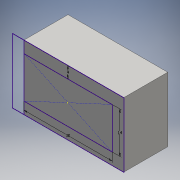
# Autodesk Inventor part: Solenoid Mount
Saved by Autodesk Inventor 2016 (Build 200138000, 138)
## iProperties
Created: 2016-05-08
Part Number: Solenoid Mount
Material: Generic
Document SubType Name: Modeling
Designer: Kenneth Daniel
Density: 1 g/cm^3
Appearance: Default
Author: Kenneth Daniel
Autodesk Inventor part; units mm, degrees
ref_plane "YZ Plane" through (0, 0, 0) normal (1, 0, 0) x (0, 1, 0)
ref_plane "XZ Plane" through (0, 0, 0) normal (0, 1, 0) x (-1, 0, 0)
ref_plane "XY Plane" through (0, 0, 0) normal (0, 0, 1) x (1, 0, 0)
sketch "Sketch1" plane through (0, 0, 0) normal (0, 1, 0) x (-1, 0, 0)
  line L0 (-15, 7) -> (-15, -7)
  line L1 (-15, -7) -> (15, -7)
  line L2 (15, -7) -> (15, 7)
  line L3 (15, 7) -> (-15, 7)
  line L4 (-15, 7) -> (15, -7) construction
  line L5 (-15, -7) -> (15, 7) construction
  line L6 (-19, 11) -> (-19, -11)
  line L7 (-19, -11) -> (19, -11)
  line L8 (19, -11) -> (19, 11)
  line L9 (19, 11) -> (-19, 11)
  line L10 (15, 7) -> (15, 11)
  line L11 (15, -7) -> (15, -11)
  point P0 (0, 0)
  dimension "d0" = 14
  dimension "d1" = 30
  dimension "d2" = 4
  constraints: 24 end point, 4 parallel, 3 perpendicular, 3 point on line, 2 midpoint, 1 vertical, 3 other
  measures "d0" distance of L0.start L0.end
  measures "d1" distance of L1.end L0.end
  measures "d2" distance between parallel lines of L3 L9
extrude "Extrusion1" add sketch "Sketch1" along normal blind 15 contours L0 L1 L11 L7 L6 L9 L10 L3
extrude "Extrusion2" add sketch "Sketch1" along normal blind 4 contours L3 L2 L1 L0
body "Solid1"
